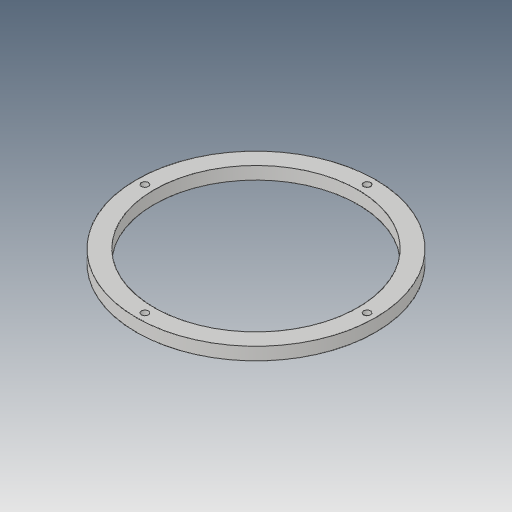
# Autodesk Inventor part: ベアリング_145mm_inside
Saved by Autodesk Inventor 2019 (Build 230136000, 136)
## iProperties
Created: 2020-10-27
Part Number: ベアリング_145mm_inside
Material: 一般
Document SubType Name: Modeling
Designer: X1 Carbon
Density: 1 g/cm^3
Appearance: 既定
Mass: 54.9582 g
Surface Area: 216.848 cm^2
Volume: 54.9582 cm^3
Author: X1 Carbon
Autodesk Inventor part; units mm, degrees
ref_plane "YZ Plane" through (0, 0, 0) normal (1, 0, 0) x (0, 1, 0)
ref_plane "XZ Plane" through (0, 0, 0) normal (0, 1, 0) x (-1, 0, 0)
ref_plane "XY Plane" through (0, 0, 0) normal (0, 0, 1) x (1, 0, 0)
sketch "スケッチ1" plane through (0, 0, 0) normal (0, 1, 0) x (-1, 0, 0)
  circle A0 centre (0, 0) radius 72.5
  circle A1 centre (0, 0) radius 85
  circle A2 centre (79, 0) radius 2.5
  circle A3 centre (-79, 0) radius 2.5
  circle A4 centre (0, 79) radius 2.5
  circle A5 centre (0, -79) radius 2.5
  dimension "d0" = 145
  dimension "d1" = 170
  dimension "d2" = 5
  dimension "d3" = 5
  dimension "d4" = 5
  dimension "d5" = 5
  constraints: 6 centre point, 2 coincident
  measures "d0" diameter of A0
  measures "d1" diameter of A1
  measures "d2" diameter of A2
  measures "d3" diameter of A3
  measures "d4" diameter of A4
  measures "d5" diameter of A5
extrude "押し出し1" add sketch "スケッチ1" along normal blind 9
